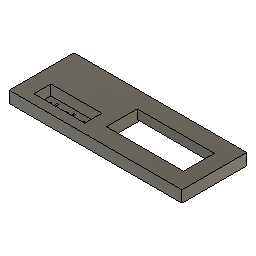
screen plate v3 (Autodesk Fusion 360 design; units mm, degrees)
Autodesk Fusion 360 part; units mm, degrees
sketch "Sketch1" plane through (0, 0, 0) normal (0, 0, 1) x (1, 0, 0)
  line L0 (112, 42) -> (-112, 42)
  line L1 (-112, 42) -> (-112, -42)
  line L2 (-112, -42) -> (112, -42)
  line L3 (112, -42) -> (112, 42)
  line L4 (112, 42) -> (-112, -42) construction
  line L5 (-112, 42) -> (112, -42) construction
  line L6 (-8, 30) -> (92, 30)
  line L7 (92, 30) -> (92, -30)
  line L8 (92, -30) -> (-8, -30)
  line L9 (-8, -30) -> (-8, 30)
  line L10 (-8, 30) -> (92, -30) construction
  line L11 (92, 30) -> (-8, -30) construction
  line L12 (92, 20) -> (-8, 20)
  line L13 (-8, 20) -> (-8, -20)
  line L14 (-8, -20) -> (92, -20)
  line L15 (92, -20) -> (92, 20)
  line L16 (92, 20) -> (-8, -20) construction
  line L17 (-8, 20) -> (92, -20) construction
  line L18 (92, 42) -> (92, -42) construction
  line L19 (-81, -19) -> (-78.46, -19) construction
  line L20 (-81, -13.92) -> (-81, -19) construction
  circle A0 centre (-75.92, -19) radius 0.85
  line L21 (-81, -16.46) -> (-81, -19) construction
  line L22 (-84.81, -19) -> (-84.81, -16.46) construction
  line L23 (-78.46, -13.92) -> (-81, -13.92) construction
  circle A1 centre (-78.46, -13.92) radius 1.25
  circle A2 centre (-86.08, -19) radius 0.85
  circle A3 centre (-81, -19) radius 2
  circle A4 centre (-84.81, -16.46) radius 1.25
  line L24 (-78.46, -19) -> (-78.46, -13.92) construction
  line L25 (-81, -19) -> (-75.92, -19) construction
  line L26 (-81, -19) -> (-84.81, -19) construction
  line L27 (-84.81, -16.46) -> (-81, -16.46) construction
  line L28 (-70, -8) -> (-92, -8)
  line L29 (-92, -8) -> (-92, -30)
  line L30 (-92, -30) -> (-70, -30)
  line L31 (-70, -30) -> (-70, -8) construction
  line L32 (-70, -8) -> (-92, -30) construction
  line L33 (-92, -8) -> (-70, -30) construction
  circle A5 centre (-53.92, -19) radius 0.85
  line L34 (-56.46, -19) -> (-56.46, -13.92) construction
  circle A6 centre (-64.08, -19) radius 0.85
  circle A7 centre (-62.81, -16.46) radius 1.25
  line L35 (-59, -16.46) -> (-59, -19) construction
  line L36 (-48, -30) -> (-48, -8) construction
  line L37 (-59, -19) -> (-53.92, -19) construction
  line L38 (-70, -8) -> (-48, -30) construction
  line L39 (-56.46, -13.92) -> (-59, -13.92) construction
  line L40 (-70, -8) -> (-70, -30) construction
  circle A8 centre (-56.46, -13.92) radius 1.25
  circle A9 centre (-59, -19) radius 2
  line L41 (-59, -19) -> (-56.46, -19) construction
  line L42 (-48, -8) -> (-70, -8)
  line L43 (-59, -13.92) -> (-59, -19) construction
  line L44 (-48, -8) -> (-70, -30) construction
  line L45 (-70, -30) -> (-48, -30)
  line L46 (-62.81, -19) -> (-62.81, -16.46) construction
  line L47 (-59, -19) -> (-62.81, -19) construction
  line L48 (-62.81, -16.46) -> (-59, -16.46) construction
  circle A10 centre (-31.92, -19) radius 0.85
  line L49 (-34.46, -19) -> (-34.46, -13.92) construction
  circle A11 centre (-42.08, -19) radius 0.85
  circle A12 centre (-40.81, -16.46) radius 1.25
  line L50 (-37, -16.46) -> (-37, -19) construction
  line L51 (-26, -30) -> (-26, -8)
  line L52 (-37, -19) -> (-31.92, -19) construction
  line L53 (-48, -8) -> (-26, -30) construction
  line L54 (-34.46, -13.92) -> (-37, -13.92) construction
  line L55 (-48, -8) -> (-48, -30) construction
  circle A13 centre (-34.46, -13.92) radius 1.25
  circle A14 centre (-37, -19) radius 2
  line L56 (-37, -19) -> (-34.46, -19) construction
  line L57 (-26, -8) -> (-48, -8)
  line L58 (-37, -13.92) -> (-37, -19) construction
  line L59 (-26, -8) -> (-48, -30) construction
  line L60 (-48, -30) -> (-26, -30)
  line L61 (-40.81, -19) -> (-40.81, -16.46) construction
  line L62 (-37, -19) -> (-40.81, -19) construction
  line L63 (-40.81, -16.46) -> (-37, -16.46) construction
  line L64 (-92, -30) -> (-112, -30) construction
  line L65 (-112, -30) -> (-112, -42) construction
  line L66 (-112, -42) -> (-92, -42) construction
  line L67 (-92, -42) -> (-92, -30) construction
  point P0 (42, 0)
  point P1 (42, 0)
  point P2 (-81, -19)
  point P3 (-81, -19)
  point P4 (-81, -19)
  point P5 (-59, -19)
  point P6 (-59, -19)
  point P7 (-59, -19)
  point P8 (-37, -19)
  point P9 (-37, -19)
  point P10 (-37, -19)
  dimension "d1" = 224
  dimension "d2" = 84
  dimension "d3" = 100
  dimension "d4" = 60
  dimension "d5" = 100
  dimension "d6" = 40
  dimension "d7" = 4
  dimension "d8" = 5.08
  dimension "d9" = 1.7
  dimension "d10" = 2.54
  dimension "d11" = 5.08
  dimension "d12" = 2.5
  dimension "d13" = 3.81
  dimension "d14" = 2.54
  dimension "d15" = 2.5
  dimension "d16" = 22
  dimension "d17" = 22
  dimension "d20" = 44
  dimension "d21" = 0
  dimension "d22" = 20
  dimension "d23" = 12
  dimension "d24" = 20
  constraint horizontal L0
  constraint perpendicular L0 L1
  constraint parallel L0 L2
  constraint parallel L1 L3
  constraint coincident L4 origin
  constraint coincident L5 origin
  constraint horizontal L6
  constraint perpendicular L6 L7
  constraint parallel L6 L8
  constraint parallel L7 L9
  constraint coincident L10 P1
  constraint coincident L11 P1
  constraint horizontal L12
  constraint perpendicular L12 L13
  constraint parallel L12 L14
  constraint parallel L13 L15
  constraint coincident L16 P1
  constraint coincident L17 P1
  constraint coincident P1 P0
  constraint coincident L0 L18.start
  constraint coincident L2 L18.end
  constraint perpendicular L2 L18
  constraint midpoint L7 L18
  constraint coincident P4 P3
  constraint horizontal L25
  constraint coincident A0.centre L25.end
  constraint horizontal L19
  constraint vertical L24
  constraint horizontal L23
  constraint vertical L20
  constraint coincident L23.start A1.centre
  constraint horizontal L26
  constraint vertical L22
  constraint horizontal L27
  constraint vertical L21
  constraint coincident L22.end A4.centre
  constraint symmetric L20 A0 A2
  constraint horizontal L28
  constraint perpendicular L28 L29
  constraint parallel L28 L30
  constraint parallel L29 L31
  constraint coincident L32 P4
  constraint coincident L33 P4
  constraint horizontal L64
  constraint vertical L65
  constraint horizontal L66
  constraint vertical L67
  measures "d1" distance of L1.end L2.end
  measures "d2" distance of L0.end L1.end
  measures "d3" distance of L7.end L8.end
  measures "d4" distance of L6.end L7.end
  measures "d5" distance of L13.end L14.end
  measures "d6" distance of L12.end L13.end
  measures "d7" diameter of A3
  measures "d8" distance of P4 A0.centre
  measures "d9" diameter of A0
  measures "d10" distance of P4 L19.end
  measures "d11" distance of P4 L20.start
  measures "d12" diameter of A1
  measures "d13" distance of P4 L22.start
  measures "d14" distance of P4 L21.start
  measures "d15" diameter of A4
  measures "d16" distance of L29.end L30.end
  measures "d17" distance of L28.end L29.end
  measures "d22" distance of L29.end L64.end
  measures "d23" distance of L29.end L66.end
  measures "d24" distance of L3 L18
extrude "Extrude1" add sketch "Sketch1" along normal blind 15 contours L0 L1 L2 L3
extrude "Extrude2" add sketch "Sketch1" along normal blind 1.5 contours L28 L29 L30 L42 L45 L51 L57 L60
extrude "Extrude3" add sketch "Sketch1" against normal blind 12 from surface at 15 contours L6 L7 L9 L12 | L7 L8 L9 L14
